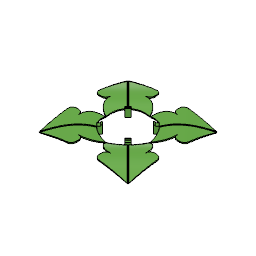
Cattail Leaves (Autodesk Fusion 360 design; units mm, degrees)
part number: 2026-05-22-17-58-27-490
Autodesk Fusion 360 part; units mm, degrees
sketch "Sketch1" plane through (0, 0, 0) normal (0, 1, 0) x (1, 0, 0)
  line L0 (67.1751, 53.033) -> (53.033, 67.1751)
  line L1 (-56.5685, 56.5685) -> (-49.4975, 63.6396)
  line L2 (-63.6396, 49.4975) -> (-67.1751, 53.033)
  line L3 (61.8637, 76.0058) -> (49.4975, 63.6396)
  line L4 (76.0058, 61.8637) -> (63.6396, 49.4975)
  line L5 (56.5685, 56.5685) -> (49.4975, 63.6396)
  line L6 (-61.8637, 76.0058) -> (-49.4975, 63.6396)
  line L7 (56.5685, 56.5685) -> (63.6396, 49.4975)
  line L8 (63.6396, 49.4975) -> (67.1751, 53.033)
  line L9 (-67.1751, 53.033) -> (-53.033, 67.1751)
  line L10 (-76.0058, 61.8637) -> (-63.6396, 49.4975)
  line L11 (-56.5685, 56.5685) -> (-63.6396, 49.4975)
  line L12 (49.4975, -63.6396) -> (53.033, -67.1751)
  line L13 (49.4975, -63.6396) -> (61.8637, -76.0058)
  line L14 (53.033, -67.1751) -> (67.1751, -53.033)
  line L15 (-63.6396, -49.4975) -> (-76.0058, -61.8637)
  line L16 (-67.1751, -53.033) -> (-53.033, -67.1751)
  line L17 (-63.6396, -49.4975) -> (-67.1751, -53.033)
  line L18 (49.4975, -63.6396) -> (63.6396, -49.4975)
  line L19 (63.6396, -49.4975) -> (76.0058, -61.8637)
  line L20 (-49.4975, -63.6396) -> (-61.8637, -76.0058)
  circle A0 centre (0, 0) radius 98
  line L21 (-56.5685, -56.5685) -> (-49.4975, -63.6396)
  line L22 (-56.5685, -56.5685) -> (-63.6396, -49.4975)
  line L23 (0, 50) -> (0, 98)
  line L24 (0, -50) -> (0, -98)
  line L25 (148, -65) -> (148, -70)
  line L26 (0, -98) -> (0, -83)
  line L27 (65, -148) -> (70, -148)
  line L28 (168, -50) -> (178, -50)
  line L29 (50, -168) -> (50, -178)
  line L30 (70, -198) -> (198, -198)
  line L31 (198, -198) -> (198, -70)
  arc A1 (148, -65) -> (97.9844, -1.7507) centre (83, -65) ccw
  arc A2 (168, -50) -> (148, -70) centre (168, -70) ccw
  arc A3 (198, -70) -> (178, -50) centre (178, -70) ccw
  arc A4 (1.7507, -97.9844) -> (65, -148) centre (65, -83) ccw
  arc A5 (70, -148) -> (50, -168) centre (70, -168) ccw
  arc A6 (50, -178) -> (70, -198) centre (70, -178) ccw
  line L32 (69.2965, -69.2965) -> (130, -130)
  line L33 (130, -130) -> (148, -70)
  line L34 (130, -130) -> (70, -148)
  line L35 (69.2965, -69.2965) -> (130, -130)
  line L36 (0, 0) -> (83, 0) construction
  line L37 (98, 0) -> (100, 0) construction
  circle A7 centre (0, 0) radius 50
  line L38 (50, 0) -> (98, 0)
  line L39 (130, -130) -> (198, -198)
  point P0 (148, 0)
  point P1 (148, -50)
  point P2 (0, -148)
  point P3 (50, -148)
  point P4 (198, -50)
  point P5 (50, -198)
  dimension "d1" = 10
  dimension "d2" = 10
  dimension "d3" = 10
  dimension "d4" = 10
  dimension "d5" = 10
  dimension "d6" = 10
  dimension "d7" = 5
  dimension "d8" = 5
  dimension "d9" = 5
  dimension "d10" = 5
  dimension "d11" = 196
  dimension "d13" = 50
  dimension "d14" = 50
  dimension "d15" = 50
  dimension "d16" = 50
  dimension "d17" = 50
  dimension "d18" = 65
  dimension "d19" = 20
  dimension "d20" = 20
  dimension "d21" = 65
  dimension "d22" = 20
  dimension "d23" = 20
  dimension "d24" = 100
  constraint coincident A0.centre L36.start
  constraint horizontal L36
  constraint perpendicular L18 L19
  constraint perpendicular L12 L18
  constraint coincident L14.end L19
  constraint perpendicular L14 L19
  constraint perpendicular L17 L22
  constraint coincident L16.end L20
  constraint perpendicular L16 L20
  constraint perpendicular L2 L11
  constraint coincident L9.end L6
  constraint perpendicular L6 L9
  constraint perpendicular L7 L8
  constraint coincident L0.end L3
  constraint perpendicular L0 L3
  constraint coincident A0 L19.end
  constraint coincident A0 L13.end
  constraint coincident A0 L4.start
  constraint coincident A0 L3.start
  constraint coincident A0 L6.start
  constraint coincident A0 L10.start
  constraint coincident A0 L15.end
  constraint coincident A0 L20.end
  constraint coincident A0 L37.start
  constraint coincident A0 L23.end
  constraint perpendicular L23 L36
  constraint coincident A0 L24.end
  constraint perpendicular L24 L36
  constraint parallel L24 L26
  constraint perpendicular L26 L27
  constraint perpendicular L25 L28
  constraint perpendicular L27 L29
  constraint perpendicular L29 L30
  constraint perpendicular L28 L31
  constraint coincident P0 L25
  constraint tangent L25 A1
  constraint coincident P1 L25
  constraint coincident P1 L28
  constraint tangent L25 A2
  constraint tangent L28 A2
  constraint coincident P4 L28
  constraint coincident P4 L31
  constraint tangent L28 A3
  constraint tangent L31 A3
  constraint coincident P2 L26
  constraint coincident P2 L27
  constraint tangent L26 A4
  constraint tangent L27 A4
  constraint coincident P3 L27
  constraint coincident P3 L29
  constraint tangent L27 A5
  constraint tangent L29 A5
  constraint coincident P5 L29
  constraint coincident P5 L30
  constraint tangent L29 A6
  constraint tangent L30 A6
  constraint coincident A0 L32.start
  constraint collinear L36 L37
  constraint coincident A0 A1.end
  constraint coincident A0 A4.start
  constraint coincident A7 L38.start
  constraint coincident L36 L38.start
  constraint coincident A7 L24.start
  constraint coincident A7 L23.start
  constraint parallel L32 L39
  measures "d1" distance of L21.start L20.start
  measures "d2" distance of L21.start L15.start
  measures "d3" distance of L5.start L4.end
  measures "d4" distance of L5.start L3.end
  measures "d5" distance of L1.start L1.end
  measures "d6" distance of L2.start L1.start
  measures "d7" distance of L12.end L12.start
  measures "d8" distance of L16.start L15.start
  measures "d9" distance of L2.start L2.end
  measures "d10" distance of L0.start L4.end
  measures "d11" diameter of A0
  measures "d13" distance of P0 P1
  measures "d14" distance of L24.end P2
  measures "d15" distance of P2 P3
  measures "d16" distance of P1 P4
  measures "d17" distance of P3 P5
  measures "d18" radius of A1
  measures "d19" radius of A2
  measures "d20" radius of A3
  measures "d21" radius of A4
  measures "d22" radius of A5
  measures "d23" radius of A6
  measures "d24" diameter of A7
extrude "Extrude1" add sketch "Sketch1" along normal blind 10 contours L12 L13 L18 L19 A0 L24 L26 A7 L38 makes body 1
ref_plane "WorkPlane1" through (0, 12.125, 0) normal (0.707107, 0, 0.707107) x (0, 1, 0)
extrude "Extrude2" add sketch "Sketch1" along normal blind 35 contours L12 L13 L14 L18 L19 bodies 1
extrude "Extrude3" add sketch "Sketch1" along normal blind 30 contours L13 L14 L19 A0 bodies 1
extrude "Extrude4" add sketch "Sketch1" along normal blind 10 contours A0 L25 A1 L32 L33 L35 bodies 1
fillet "Fillet1" radius 2.5 tangency weight 0.25 1 edges at (99.6482, 10, 99.6482) on bodies 1
extrude "Extrude5" add sketch "Sketch1" along normal blind 10 contours A0 L27 A4 L32 L34 L35 bodies 1
extrude "Extrude6" add sketch "Sketch1" along normal blind 10 contours L28 L31 A2 A3 L33 L39 | L29 L30 A5 A6 L34 L39 bodies 1
fillet "Fillet2" radius 2.5 1 edges at (99.6482, 10, 99.6482) on bodies 1
delete_body "RemoveBody1" bodies 1
ref_plane "WorkPlane2" through (0, 12.125, 0) normal (-0.707107, 0, 0.707107) x (0, 1, 0)
sketch "Sketch2" plane through (0, 0, 0) normal (-0.707107, 0, 0.707107) x (0, 1, 0)
  spline S0 degree 5 poles (0, -50) (2.3282, -53.9773) (6.7753, -61.9879) (12.8185, -74.1716) (19.6004, -90.7577) (25.8127, -112.0961) (29.5782, -134.089) (30.7299, -156.781) (29.2366, -180.1804) (25.2618, -204.2435) (19.0192, -228.9131) (12.3722, -249.0909) (6.5184, -264.4566) (2.2361, -274.8019) (0, -280) knots 0 0 0 0 0 0 0.1 0.2 0.3 0.4 0.5 0.6 0.7 0.8 0.9 1 1 1 1 1 1
  line L0 (0, -50) -> (0, -55)
  line L1 (0, -280) -> (0, -275)
  spline S1 degree 5 poles (0, -55) (1.9432, -58.7848) (5.6548, -66.4099) (10.6975, -78.0135) (16.3543, -93.8228) (21.5318, -114.1838) (24.6649, -135.1919) (25.6157, -156.8909) (24.3626, -179.2876) (21.0442, -202.3381) (15.8399, -225.9856) (10.3024, -245.3386) (5.4274, -260.0819) (1.8617, -270.0106) (0, -275) knots 0 0 0 0 0 0 0.1 0.2 0.3 0.4 0.5 0.6 0.7 0.8 0.9 1 1 1 1 1 1
  point P0 (30, -150)
  point P1 (25, -150)
  constraint vertical L0
  constraint vertical L1
extrude "Extrude7" add sketch "Sketch2" along normal blind 100 separate body makes body 2
extrude "Extrude8" add 1 faces at (112.3319, 26.3904, 112.3319) along direction (0.707107, 0, -0.707107) blind 100 on bodies 2 bodies 2
extrude "Extrude9" cut sketch "Sketch1" along normal blind 40 contours A0 L25 A1 L32 L33 L35 keep common part bodies 2
fillet "Fillet3" radius 2.5 1 edges at (99.3815, 29.51, 99.3815) on bodies 2
extrude "Extrude10" add sketch "Sketch2" along normal blind 110 separate body makes body 3
extrude "Extrude11" cut sketch "Sketch1" along normal blind 50 contours A0 L27 A4 L32 L34 L35 | L29 L30 A5 A6 L34 L39 keep common part bodies 3
fillet "Fillet4" radius 2.5 1 edges at (130.3441, 28.1262, 130.3441) on bodies 3
delete_body "RemoveBody2" bodies 2
extrude "Extrude12" add sketch "Sketch2" against normal blind 120 separate body makes body 4
extrude "Extrude13" cut sketch "Sketch1" along normal blind 40 contours A0 L25 A1 L32 L33 L35 | L28 L31 A2 A3 L33 L39 keep common part bodies 4
fillet "Fillet5" radius 2.5 1 edges at (130.3441, 28.1262, 130.3441) on bodies 4
extrude "Extrude14" add sketch "Sketch1" along normal blind 30 contours L13 L14 L19 A0 bodies 3 4
extrude "Extrude15" add sketch "Sketch1" along normal blind 35 contours L12 L13 L14 L18 L19 bodies 3
extrude "Extrude16" add 1 faces at (63.9417, 30, 62.3679) along direction (0, 1, 0) blind 10 on bodies 3 bodies 3
extrude "Extrude17" add 1 faces at (56.5685, 35, 61.2826) along direction (0, 1, 0) blind 10 on bodies 3 bodies 3
extrude "Extrude18" add 1 faces at (63.9417, 40, 62.3679) along direction (0, 1, 0) blind 10 on bodies 3 bodies 3
extrude "Extrude19" add 1 faces at (56.5685, 45, 61.2826) along direction (0, 1, 0) blind 10 on bodies 3 bodies 3
mirror "Mirror1" about plane through (0, 12.125, 0) normal (0.707107, 0, 0.707107) of bodies 3 makes body 5
mirror "Mirror2" about plane through (0, 0, 0) normal (0, 0, 1) of bodies 3 makes body 6
mirror "Mirror3" about plane through (0, 0, 0) normal (1, 0, 0) of bodies 3 makes body 7
extrude "Extrude20" cut 4 faces at (63.9417, 50, -62.3679) (63.9417, 50, 62.3679) (-63.9417, 50, 62.3679) (-62.3679, 50, -63.9417) along direction (0, -1, 0) blind 10 on bodies 3 5 6 7 bodies 3 5 6 7
extrude "Extrude21" cut 1 faces at (63.9417, 40, 62.3679) along direction (0, -1, 0) blind 10 on bodies 3 bodies 3
extrude "Extrude22" cut 1 faces at (-63.9417, 40, 62.3679) along direction (0, -1, 0) blind 10 on bodies 7 bodies 7
extrude "Extrude23" cut 2 faces at (63.9417, 40, -62.3679) (-62.3679, 40, -63.9417) along direction (0, -1, 0) blind 10 on bodies 5 6 bodies 5 6
extrude "Extrude24" cut 4 faces at (56.5685, 55, 61.2826) (56.5685, 55, -61.2826) (-61.2826, 55, -56.5685) (-56.5685, 55, 61.2826) along direction (0, -1, 0) blind 20 on bodies 3 5 6 7 bodies 3 5 6 7
